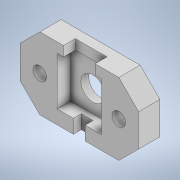
# Autodesk Inventor part: ポテンショメータホルダ
Saved by Autodesk Inventor 2021.3 (Build 253353000, 353)
## iProperties
Created: 2022-04-18
Part Number: ポテンショメータホルダ
Material: 一般
Document SubType Name: Modeling
Designer: gilte
Density: 1 g/cm^3
Appearance: 既定
Author: gilte
## iProperties of the stored document _3D プリント.ipt
Created: 2022-04-18
Part Number: _3D プリント
Material: 一般
Document SubType Name: Modeling
Designer: gilte
Density: 1 g/cm^3
Appearance: 既定
Author: gilte
Autodesk Inventor part; units mm, degrees
ref_plane "YZ Plane" through (0, 0, 0) normal (1, 0, 0) x (0, 1, 0)
ref_plane "XZ Plane" through (0, 0, 0) normal (0, 1, 0) x (-1, 0, 0)
ref_plane "XY Plane" through (0, 0, 0) normal (0, 0, 1) x (1, 0, 0)
sketch "スケッチ1" plane through (0, 0, 0) normal (0, 0, 1) x (1, 0, 0)
  line L0 (0, 0) -> (11.2, 0)
  line L1 (11.2, 0) -> (11.2, 12.2)
  line L2 (11.2, 12.2) -> (0, 12.2)
  line L3 (0, 12.2) -> (0, 0)
  line L4 (-9.4, -3.5) -> (20.6, -3.5)
  line L5 (20.6, -3.5) -> (20.6, 14.7)
  line L6 (20.6, 14.7) -> (-9.4, 14.7)
  line L7 (-9.4, 14.7) -> (-9.4, -3.5)
  dimension "d0" = 11.2
  dimension "d1" = 12.2
  dimension "d2" = 2.5
  dimension "d3" = 3.5
  dimension "d4" = 9.4
  dimension "d5" = 9.4
  constraints: 16 end point, 4 parallel, 2 horizontal, 2 perpendicular
  measures "d0" distance of L2.end L1.end
  measures "d1" distance of L0.end L1.end
  measures "d2" distance between parallel lines of L6 L2
  measures "d3" distance between parallel lines of L4 L0
  measures "d4" distance between parallel lines of L7 L3
  measures "d5" distance between parallel lines of L5 L1
extrude "押し出し1" add sketch "スケッチ1" along normal blind 3.4
extrude "押し出し2" add sketch "スケッチ1" against normal blind 2 contours L3 L2 L1 L0 | L7 L6 L5 L4
sketch "スケッチ2" plane through (0, 0, 3.4) normal (0, 0, 1) x (1, 0, 0)
  line L0 (11.2, 0) -> (0, 0) projected
  line L1 (0, 12.2) -> (11.2, 12.2) projected
  point P0 (5.6, 5.6)
  dimension "d41" = 6.6
  measures "d41" distance from line of L1 point (5.6, 5.6)
hole "穴1" at (5.6, 5.6, 3.4) direction (0, 0, -1) diameter 6 end through all
sketch "スケッチ3" plane through (0, 0, 3.4) normal (0, 0, 1) x (1, 0, 0)
  line L0 (0, 12.2) -> (11.2, 12.2) projected
  line L1 (-9.4, 14.7) -> (20.6, 14.7) projected
  line L2 (9.6, 12.2) -> (1.6, 12.2)
  line L3 (1.6, 12.2) -> (1.6, 14.7)
  line L4 (1.6, 14.7) -> (9.6, 14.7)
  line L5 (9.6, 14.7) -> (9.6, 12.2)
  line L6 (-9.4, 14.7) -> (-9.4, -3.5) projected
  line L7 (20.6, -3.5) -> (20.6, 14.7) projected
  point P0 (0, 0)
  point P1 (9.6, 14.7)
  dimension "d17" = 8
  dimension "d18" = 11
  dimension "d33" = 30
  constraints: 8 end point, 2 parallel, 2 point on line, 1 horizontal, 1 perpendicular
  measures "d17" distance of L3.end L4.end
  measures "d18" distance between parallel lines of L6 L3
  measures "d33" distance between parallel lines of L6 L7
extrude "押し出し3" cut sketch "スケッチ3" against normal blind 3
sketch "スケッチ4" plane through (0, 0, -2) normal (0, 0, -1) x (-1, 0, 0)
  circle A0 centre (-5.6, 5.6) radius 3 projected
  line L0 (-20.6, -3.5) -> (9.4, -3.5) projected
  line L1 (9.4, 14.7) -> (-20.6, 14.7) projected
  point P0 (0, 0)
  point P1 (-15.6, 5.6)
  point P2 (4.4, 5.6)
  dimension "d21" = 20
  dimension "d22" = 10
  dimension "d23" = 10
  dimension "d24" = 9.1
  dimension "d25" = 18.2
  measures "d21" distance of point (-15.6, 5.6) point (4.4, 5.6)
  measures "d22" distance of A0.centre point (4.4, 5.6)
  measures "d23" distance of point (-15.6, 5.6) A0.centre
  measures "d24" distance from line of L0 point (4.4, 5.6)
  measures "d25" distance between parallel lines of L1 L0
hole "穴2" at (15.6, 5.6, -2) at (-4.4, 5.6, -2) direction (0, 0, 1) diameter 3.4 end through all
sketch "スケッチ5" plane through (0, 0, 3.4) normal (0, 0, 1) x (1, 0, 0)
  line L0 (20.6, -3.5) -> (-9.4, -3.5) projected
  line L1 (11.2, 0) -> (0, 0) projected
  line L2 (7.1, -3.5) -> (4.1, -3.5)
  line L3 (4.1, -3.5) -> (4.1, 0)
  line L4 (4.1, 0) -> (7.1, 0)
  line L5 (7.1, 0) -> (7.1, -3.5)
  line L6 (-9.4, 14.7) -> (-9.4, -3.5) projected
  point P0 (7.1, 0)
  dimension "d34" = 3
  dimension "d35" = 13.5
  constraints: 8 end point, 2 parallel, 2 point on line, 1 horizontal, 1 perpendicular
  measures "d34" distance of L3.end L4.end
  measures "d35" distance between parallel lines of L6 L3
extrude "押し出し4" cut sketch "スケッチ5" against normal blind 2
chamfer "面取り1" distance 5 angle 45 4 edges at (20.6, -3.5, 0.7) (20.6, 14.7, 0.7) (-9.4, -3.5, 0.7) (-9.4, 14.7, 0.7)
equation "\"d24\" = 0.5 * d25"
